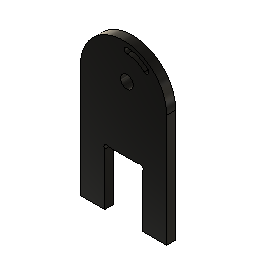
CameraTowerNew v2 (Autodesk Fusion 360 design; units mm, degrees)
Autodesk Fusion 360 part; units mm, degrees
sketch "Sketch1" plane through (0, 0, 0) normal (0, 1, 0) x (1, 0, 0)
  line L0 (46, -60) -> (0, -60) construction
  line L1 (0, -60) -> (0, 0)
  line L2 (13, 0) -> (13, -27.8787)
  line L3 (15.1213, -30) -> (30.8787, -30)
  line L4 (33, -27.8787) -> (33, 0)
  line L5 (0, 0) -> (13, 0)
  line L6 (33, 0) -> (46, 0)
  line L7 (13, 0) -> (33, 0) construction
  line L8 (56.7697, -71.289) -> (65.8307, -94.5891) construction
  line L9 (56.7697, -71.289) -> (33.4695, -80.3499) construction
  line L10 (46, 0) -> (46, -60)
  line L11 (42.5305, -103.6501) -> (65.8307, -94.5891) construction
  line L12 (13, -30) -> (14.0607, -28.9393) construction
  line L13 (33, -30) -> (31.9393, -28.9393) construction
  arc A0 (13, -27.8787) -> (15.1213, -30) centre (14.0607, -28.9393) ccw
  arc A1 (15.1213, -30) -> (13, -27.8787) centre (14.0607, -28.9393) ccw construction
  arc A2 (30.8787, -30) -> (33, -27.8787) centre (31.9393, -28.9393) ccw
  arc A3 (33, -27.8787) -> (30.8787, -30) centre (31.9393, -28.9393) ccw construction
  line L14 (13, -27.8787) -> (13, -30) construction
  line L15 (13, -30) -> (15.1213, -30) construction
  line L16 (30.8787, -30) -> (33, -30) construction
  line L17 (33, -30) -> (33, -27.8787) construction
  line L18 (33.4695, -80.3499) -> (42.5305, -103.6501) construction
  line L19 (61.3002, -82.939) -> (38, -92) construction
  arc A4 (0, -60) -> (46, -60) centre (23, -60) ccw
  line L20 (42.5305, -103.6501) -> (38.0568, -105.3898) construction
  line L21 (38.0568, -105.3898) -> (21.7471, -63.4494) construction
  line L22 (33.4695, -80.3499) -> (26.2208, -61.7097) construction
  line L23 (21.7471, -63.4494) -> (26.2208, -61.7097) construction
  line L24 (23.4868, -67.9231) -> (27.9605, -66.1834) construction
  line L25 (23.4868, -67.9231) -> (26.2208, -61.7097) construction
  circle A5 centre (24.8538, -64.8164) radius 3.3941
  line L26 (24.8538, -64.8164) -> (30.0729, -78.2373) construction
  arc A6 (24.8538, -79.2164) -> (30.0729, -78.2373) centre (24.8538, -64.8164) ccw construction
  line L27 (24.8538, -64.8164) -> (24.8538, -79.2164) construction
  line L28 (24.8538, -64.8164) -> (35.0361, -74.9988) construction
  arc A7 (30.0729, -78.2373) -> (35.0361, -74.9988) centre (24.8538, -64.8164) ccw construction
  line L29 (24.8538, -79.2164) -> (24.8538, -80.7164) construction
  line L30 (35.0361, -74.9988) -> (36.0968, -76.0594) construction
  arc A8 (24.8538, -80.7164) -> (24.8538, -77.7164) centre (24.8538, -79.2164) ccw construction
  arc A9 (24.8538, -77.7164) -> (24.8538, -80.7164) centre (24.8538, -79.2164) ccw
  arc A10 (33.9755, -73.9381) -> (36.0968, -76.0594) centre (35.0361, -74.9988) ccw construction
  arc A11 (36.0968, -76.0594) -> (33.9755, -73.9381) centre (35.0361, -74.9988) ccw
  arc A12 (24.8538, -77.7164) -> (33.9755, -73.9381) centre (24.8538, -64.8164) ccw
  arc A13 (24.8538, -80.7164) -> (36.0968, -76.0594) centre (24.8538, -64.8164) ccw
  point P0 (61.3002, -82.939)
  point P1 (23, -60)
  point P2 (24.8538, -64.8164)
  point P3 (24.8538, -80.7164)
  point P4 (36.0968, -76.0594)
  dimension "d2" = 60
  dimension "d3" = 30
  dimension "d4" = 20
  dimension "d5" = 13
  dimension "d6" = 46
  dimension "d7" = 13
  dimension "d31" = 25
  dimension "d48" = 1.5
  dimension "d49" = 1.5
  dimension "d50" = 45
  dimension "d51" = 45
  dimension "d64" = 21.25
  dimension "d65" = 92
  dimension "d66" = 38
  dimension "d67" = 25
  dimension "d70" = 4.8
  dimension "d71" = 45
  dimension "d72" = 4.8
  dimension "d73" = 12
  dimension "d75" = 14.4
  dimension "d76" = 45
  dimension "d77" = 14.4
  dimension "d78" = 3
  dimension "d79" = 3
  dimension "d80" = 12.9
  dimension "d81" = 15.9
  constraint horizontal L5
  constraint vertical L10
  constraint horizontal L0
  constraint vertical L1
  constraint coincident L1.end L5.start
  constraint perpendicular L2 L5
  constraint perpendicular L2 L3
  constraint coincident L4.end L5
  constraint perpendicular L4 L5
  constraint midpoint L8 P0
  constraint perpendicular L8 L9
  constraint coincident L12.end A0.centre
  constraint coincident L12.start A0
  constraint coincident L13.end A2.centre
  constraint coincident L13.start A2
  constraint concentric A0 A1
  constraint concentric A2 A3
  constraint perpendicular L5 L14
  constraint perpendicular L2 L15
  constraint perpendicular L2 L16
  constraint perpendicular L5 L17
  constraint perpendicular L11 L18
  constraint coincident P0 L19.start
  constraint midpoint L18 L19.end
  constraint perpendicular L9 L18
  constraint midpoint L0 P1
  constraint coincident P1 A4.centre
  constraint perpendicular L18 L20
  constraint perpendicular L20 L21
  constraint perpendicular L9 L22
  constraint perpendicular L22 L23
  constraint coincident L21 L24.start
  constraint coincident L22 L24.end
  constraint perpendicular L22 L24
  constraint midpoint L25 P2
  constraint coincident P2 A5.centre
  constraint coincident L24.end A5
  constraint perpendicular L9 L26
  constraint vertical L27
  constraint coincident A6.start L27.end
  constraint coincident L28.end A7.end
  constraint parallel L27 L29
  constraint parallel L28 L30
  constraint coincident L27 A8.end
  constraint coincident P3 L29.end
  constraint coincident L28 A10.start
  constraint coincident P4 L30.end
  constraint concentric A8 A9
  constraint concentric A10 A11
  measures "d2" distance of L1.end L0.end
  measures "d3" distance of L2.start L12.start
  measures "d4" distance of L12.start L13.start
  measures "d5" distance of L1 L2
  measures "d6" distance of L1 L10
  measures "d7" distance of L6.end L4.end
  measures "d31" distance of L8.start L8.end
  measures "d48" distance of L12.start L12.end
  measures "d49" distance of L13.start L13.end
  measures "d50" angle of L3 L12
  measures "d51" angle of L3 L13
  measures "d64" angle of L0 L11
  measures "d65" distance of L5 L19.end
  measures "d66" distance of L1 L19.end
  measures "d67" distance of L8.start L9.end
  measures "d70" distance of L11.start L20.end
  measures "d71" distance of L20.end L21.end
  measures "d72" distance of L23 L24
  measures "d73" distance of L24 L26.end
  measures "d75" distance of P2 L28.end
  measures "d76" angle of L27 L28
  measures "d77" radius of A7
  measures "d78" diameter of A8
  measures "d79" diameter of A10
  measures "d80" radius of A12
  measures "d81" radius of A13
extrude "Extrude1" add sketch "Sketch1" along normal blind 4.8
sketch "Sketch2" plane through (0, 0, 0) normal (0, 0, -1) x (1, 0, 0)
  line L0 (13, 0) -> (0, 0)
  line L1 (0, 0) -> (0, -4.8)
  line L2 (0, -4.8) -> (13, -4.8)
  line L3 (13, -4.8) -> (13, 0)
  line L4 (46, 0) -> (33, 0)
  line L5 (33, 0) -> (33, -4.8)
  line L6 (33, -4.8) -> (46, -4.8)
  line L7 (46, -4.8) -> (46, 0)
  line L8 (0, 0) -> (13, -4.8) construction
  line L9 (33, 0) -> (46, -4.8) construction
  circle A0 centre (6.5, -2.4) radius 1.5
  circle A1 centre (39.5, -2.4) radius 1.5
  point P0 (6.5, -2.4)
  point P1 (39.5, -2.4)
  dimension "d52" = 3
  dimension "d53" = 3
  constraint coincident L0.end L1.start
  constraint coincident L2.end L3.start
  constraint coincident L4.end L5.start
  constraint coincident L6.end L7.start
  constraint midpoint L8 P0
  constraint midpoint L9 P1
  constraint coincident P0 A0.centre
  constraint coincident P1 A1.centre
  measures "d52" diameter of A0
  measures "d53" diameter of A1
extrude "Extrude2" cut sketch "Sketch2" against normal blind 8 contours A0 | A1
thread "Thread1" "ISO Metric profile 3.0 M3x0.5 6H" major diameter 3.086 minor diameter 2.529 pitch 0.5 angle 60 modelled right hand crest width 0.1368 on face at (7.9981, 2.4748, 5.3333) crest through (7.7645, 2.4, 0.125)
thread "Thread2" "ISO Metric profile 3.0 M3x0.5 6H" major diameter 3.086 minor diameter 2.529 pitch 0.5 angle 60 modelled right hand crest width 0.1368 on face at (39.9063, 0.9561, 5.3333) crest through (40.7645, 2.4, 0.125)
